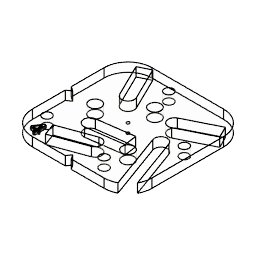
BearingPlate1_v15 (Autodesk Fusion 360 design; units mm, degrees)
Autodesk Fusion 360 part; units mm, degrees
derive "Sketch1" from "TopPlate v30"
sketch "sketch 220" plane through (0, 0, 0) normal (0, 0, 1) x (1, 0, 0)
  line L0 (55, -55) -> (-55, -55)
  line L1 (-55, -55) -> (-55, 55)
  line L2 (-55, 55) -> (55, 55)
  line L3 (55, 55) -> (55, -55)
  circle A0 centre (0, 9) radius 2
  circle A1 centre (0, -11) radius 1
  circle A2 centre (0, 0) radius 0.5
  circle A3 centre (-27, 47.000001) radius 3
  circle A4 centre (-1, 47.000001) radius 3
  circle A5 centre (46.868551, 27.224139) radius 3
  line L4 (46.998834, 0.999974) -> (46.985542, 27.034985) construction
  line L5 (-1, 47.000001) -> (-27, 47.000001) construction
  circle A6 centre (47.00084, 0.993878) radius 3
  circle A7 centre (-47.000001, -1) radius 3
  line L6 (-47.00798, -2.91748) -> (-47.001224, -28.99998) construction
  circle A8 centre (-47.000001, -27) radius 3
  circle A9 centre (0.015779, -47.131819) radius 3
  line L7 (1, -47.000001) -> (27, -47.000001) construction
  circle A10 centre (27.974555, -46.624476) radius 3
  line L8 (27.974555, -46.624476) -> (11, 0) construction
  line L9 (0, 0) -> (5, 0) construction
  line L10 (9.120675, -0.684205) -> (12.879325, 0.684205) construction
  line L11 (12.879325, 0.684205) -> (16.984556, -10.591746)
  line L12 (9.120675, -0.684205) -> (13.225906, -11.960156)
  line L13 (16.984556, -10.591746) -> (13.225906, -11.960156)
  circle A11 centre (11, 0) radius 2
  line L14 (-0.684205, -9.120675) -> (-11.960156, -13.225906)
  line L15 (-10.591746, -16.984556) -> (-11.960156, -13.225906)
  line L16 (0.684205, -12.879325) -> (-10.591746, -16.984556)
  circle A12 centre (0, -11) radius 2
  line L17 (-46.624476, -27.974555) -> (0, -11) construction
  circle A13 centre (7.778175, 7.778175) radius 2
  line L18 (7.778175, 7.778175) -> (46.868551, 27.224139) construction
  line L19 (7.778175, 7.778175) -> (8.668964, 5.987506) construction
  line L20 (8.668964, 5.987506) -> (19.412977, 11.33224)
  line L21 (19.412977, 11.33224) -> (17.631398, 14.913578)
  line L22 (17.631398, 14.913578) -> (6.887385, 9.568843)
  circle A14 centre (-7.778175, 7.778175) radius 2
  line L23 (-7.778175, 7.778175) -> (-27, 47.000001) construction
  line L24 (-7.778175, 7.778175) -> (-9.574099, 6.898028) construction
  line L25 (-9.574099, 6.898028) -> (-14.854975, 17.673572)
  line L26 (-5.982251, 8.658321) -> (-11.263127, 19.433864)
  line L27 (-11.263127, 19.433864) -> (-14.854975, 17.673572)
  line L28 (46.998834, 0.999974) -> (-6.363961, -6.363961) construction
  line L29 (0.015779, -47.131819) -> (-11, 0) construction
  line L30 (0, 9) -> (-47.00798, -2.91748) construction
  circle A15 centre (7.778175, -7.778175) radius 2
  line L31 (7.778175, -7.778175) -> (-1, 47.000001) construction
  line L32 (0, 0) -> (9, 0) construction
  circle A16 centre (-6.363961, -6.363961) radius 2
  line L33 (0, -11) -> (0.684205, -12.879325)
  circle A17 centre (-11, 0) radius 2
  line L34 (-11, 0) -> (-9.052486, 0.455178) construction
  line L35 (-9.052486, 0.455178) -> (-6.321415, -11.229908)
  line L36 (-6.321415, -11.229908) -> (-10.216444, -12.140265)
  line L37 (-10.216444, -12.140265) -> (-12.947514, -0.455178)
  line L38 (-6.363961, -6.363961) -> (-6.090557, -8.345185) construction
  line L39 (-6.090557, -8.345185) -> (5.79679, -6.704761)
  line L40 (5.79679, -6.704761) -> (5.249981, -2.742312)
  line L41 (5.249981, -2.742312) -> (-6.637365, -4.382737)
  line L42 (7.778175, -7.778175) -> (9.752979, -7.461713) construction
  line L43 (9.752979, -7.461713) -> (7.854211, 4.387113)
  line L44 (7.854211, 4.387113) -> (3.904602, 3.75419)
  line L45 (3.904602, 3.75419) -> (5.80337, -8.094636)
  line L46 (0, 9) -> (0.491492, 7.061331) construction
  line L47 (0.491492, 7.061331) -> (-11.140519, 4.11238)
  line L48 (-11.140519, 4.11238) -> (-12.123503, 7.989717)
  line L49 (-12.123503, 7.989717) -> (-0.491492, 10.938669)
  line L50 (20, -20) -> (-20, -20)
  line L51 (-20, -20) -> (-20, 20)
  line L52 (-20, 20) -> (20, 20)
  line L53 (20, 20) -> (20, -20)
  line L54 (20, -20) -> (-20, 20) construction
  line L55 (-20, -20) -> (20, 20) construction
  line L56 (15.105231, -11.275951) -> (11, 0) construction
  line L57 (13.052616, -5.637976) -> (14.931941, -4.95377) construction
  line L58 (13.052616, -5.637976) -> (11.17329, -6.322181) construction
  line L59 (14.931941, -4.95377) -> (17.281097, -4.098514) construction
  line L60 (16.767943, -2.68902) -> (17.794251, -5.508008)
  line L61 (17.794251, -5.508008) -> (9.337288, -8.586931)
  line L62 (16.767943, -2.68902) -> (8.31098, -5.767943)
  line L63 (8.31098, -5.767943) -> (9.337288, -8.586931)
  line L64 (18.522187, 13.122909) -> (7.778175, 7.778175) construction
  line L65 (13.150181, 10.450542) -> (14.04097, 8.659873) construction
  line L66 (14.04097, 8.659873) -> (15.154457, 6.421537) construction
  line L67 (13.811455, 5.753445) -> (16.497458, 7.089629)
  line L68 (13.811455, 5.753445) -> (9.802904, 13.811455)
  line L69 (9.802904, 13.811455) -> (12.488907, 15.147639)
  line L70 (12.488907, 15.147639) -> (16.497458, 7.089629)
  line L71 (-13.059051, 18.553718) -> (-7.778175, 7.778175) construction
  line L72 (-10.418613, 13.165946) -> (-6.377784, 15.146275) construction
  line L73 (-7.037894, 16.493218) -> (-5.717674, 13.799332)
  line L74 (-7.037894, 16.493218) -> (-5.717674, 13.799332) construction
  line L75 (-5.717674, 13.799332) -> (-13.799332, 9.838675)
  line L76 (-13.799332, 9.838675) -> (-15.119551, 12.532561)
  line L77 (-15.119551, 12.532561) -> (-7.037894, 16.493218)
  line L78 (0, 9) -> (-11.632011, 6.051048) construction
  line L79 (-5.816006, 7.525524) -> (-4.710149, 3.16352) construction
  line L80 (-6.16415, 2.794901) -> (-3.256147, 3.532139) construction
  line L81 (-3.256147, 3.532139) -> (-6.16415, 2.794901)
  line L82 (-6.16415, 2.794901) -> (-8.375864, 11.518909)
  line L83 (-8.375864, 11.518909) -> (-5.467861, 12.256147)
  line L84 (-5.467861, 12.256147) -> (-3.256147, 3.532139)
  line L85 (-11, 0) -> (-8.268929, -11.685087) construction
  line L86 (-9.634465, -5.842543) -> (-14.016372, -6.866695) construction
  line L87 (-14.357756, -5.406059) -> (-13.674988, -8.327331) construction
  line L88 (-14.357756, -5.406059) -> (-13.674988, -8.327331)
  line L89 (-13.674988, -8.327331) -> (-4.911173, -6.279028)
  line L90 (-4.911173, -6.279028) -> (-5.593941, -3.357756)
  line L91 (-5.593941, -3.357756) -> (-14.357756, -5.406059)
  line L92 (5.523385, -4.723536) -> (-6.363961, -6.363961) construction
  line L93 (-0.420288, -5.543749) -> (-1.035447, -1.085994) construction
  line L94 (-2.521365, -1.291047) -> (0.450471, -0.880941) construction
  line L95 (-2.521365, -1.291047) -> (0.450471, -0.880941)
  line L96 (0.450471, -0.880941) -> (1.68079, -9.796451)
  line L97 (1.68079, -9.796451) -> (-1.291047, -10.206557)
  line L98 (-1.291047, -10.206557) -> (-2.521365, -1.291047)
  line L99 (0, -11) -> (-11.275951, -15.105231) construction
  line L100 (-5.637976, -13.052616) -> (-4.098514, -17.281097) construction
  line L101 (-5.508008, -17.794251) -> (-2.68902, -16.767943) construction
  line L102 (-2.68902, -16.767943) -> (-5.508008, -17.794251)
  line L103 (-5.508008, -17.794251) -> (-8.586931, -9.337288)
  line L104 (-8.586931, -9.337288) -> (-5.767943, -8.31098)
  line L105 (-5.767943, -8.31098) -> (-2.68902, -16.767943)
  line L106 (7.778175, -7.778175) -> (5.879406, 4.070651) construction
  line L107 (6.82879, -1.853762) -> (11.2721, -1.141723) construction
  line L108 (11.034754, 0.33938) -> (11.509446, -2.622827) construction
  line L109 (11.034754, 0.33938) -> (11.509446, -2.622827)
  line L110 (11.509446, -2.622827) -> (2.622827, -4.046903)
  line L111 (2.622827, -4.046903) -> (2.148135, -1.084696)
  line L112 (2.148135, -1.084696) -> (11.034754, 0.33938)
  line L113 (0, -20) -> (0, -18.5) construction
  line L114 (0, -20) -> (1, -20) construction
  line L115 (0, -20) -> (-1, -20) construction
  line L116 (-1, -20) -> (0, -18.5)
  line L117 (1, -20) -> (0, -18.5)
  line L118 (-20, 0) -> (-18.5, 0) construction
  line L119 (-18.5, 0) -> (-20, 1)
  line L120 (-18.5, 0) -> (-20, -1)
  line L121 (-20, -1) -> (-20, 0) construction
  line L122 (-20, 0) -> (-20, 1) construction
  circle A18 centre (6, -14) radius 1.5
  circle A19 centre (16.104187, 2.735059) radius 1.5
  circle A20 centre (-2.329709, 15.997455) radius 1.5
  circle A21 centre (-15.675516, -11.444861) radius 1.5
  line L123 (-15.271796, -18.277941) -> (-12.271824, -18.255298) construction
  line L124 (-12.271824, -18.255298) -> (-12.301745, -14.291027) construction
  line L125 (-12.301745, -14.291027) -> (-15.301717, -14.313669) construction
  line L126 (-15.301717, -14.313669) -> (-15.271796, -18.277941) construction
extrude "Extrude1" add sketch "sketch 220" along normal blind 3 contours A0 | A0 L47 L49 L84 | A14 L26 L47 L49 L82 L84 | L26 L49 L83 L84 | L47 L81 L82 L84 | A14 L26 L49 L82 L83 | A14 L26 L49 | A14 L25 L47 L48 L49 L82 | A14 L49 L82 | A14 L25 L26 L49 L75 L82 L83 | A14 L49 L82 | A14 L49 L82 | L25 L26 L75 L77 | L26 L73 L75 L77 | A14 L49 L82 | A14 L25 L49 | L25 L26 L27 L77 | L25 L75 L76 L77 | A1 L97 | A1 A12 L33 L97 | A1 L97 | A1 A12 L97 L98 | A1 A12 L33 L97 L98 | L14 A12 L39 L96 L97 L98 | L14 L16 A12 L98 L105 | L14 A12 L98 | L16 L102 L103 L105 | L14 L16 L35 L36 L103 L105 | L14 A16 L35 L39 L98 L104 L105 | L39 L41 L45 L96 L110 L111 | L39 L41 L96 L98 | L14 L15 L16 L103 | L14 L35 L104 L105 | A16 L39 L41 L90 L98 | L39 L40 L45 L110 | A15 L39 L40 L43 L45 L62 L63 L110 | L41 L95 L96 L98 | L14 L36 L103 | L14 L35 L36 | L14 L35 L36 L103 L104 | A16 L35 L89 L90 | L41 L45 L110 L111 | L40 L41 L45 L110 | A15 L61 L63 | L41 L45 L111 L112 | A16 L35 L36 L37 L89 L103 L104 | A16 L35 L89 | A16 L41 L90 | A16 L35 L41 L90 L91 | L40 L41 L43 L45 L110 L112 | A15 L43 L62 L63 | A15 L61 L63 | L12 A15 L43 L61 L62 | A16 L35 L89 L90 | A16 L35 L37 L89 L91 | A16 L35 L89 | L12 L43 L62 L110 | L12 A11 L43 L110 L112 | L43 L44 L45 L112 | L11 L12 L13 L61 | L11 L12 L61 L62 | L37 L88 L89 L91 | A17 L35 L37 L91 | L11 L12 A11 L62 L109 L110 | L12 A11 L109 L110 | L11 L60 L61 L62 | A17 | A11 L109 L112 | A11 L109 L112 | A13 | A13 L20 L22 L68 | L22 L68 L69 L70 | L20 L22 L68 L70 | L20 L67 L68 L70 | L20 L21 L22 L70 | L50 L51 L52 L53 L116 L117 L119 L120 picked at (-1.219323, 9.210669) picked at (-3.564662, 8.147682) picked at (-4.838382, 7.931269) picked at (-6.443705, 11.149054) picked at (-5.399604, 3.848426) picked at (-7.839618, 11.011821) picked at (-6.458435, 9.358913) picked at (-10.94604, 6.333375) picked at (-7.145501, 7.044572) picked at (-9.614425, 10.627606) picked at (-7.781251, 9.547253) picked at (-7.864423, 6.890387) picked at (-11.237291, 13.321545) picked at (-7.654351, 13.963839) picked at (-7.962534, 9.534137) picked at (-9.927706, 8.286734) picked at (-11.140191, 16.153214) picked at (-12.742802, 11.470092) picked at (-0.071212, -10.70625) picked at (0.694181, -12.511167) picked at (-0.087629, -10.031035) picked at (-0.953643, -9.889262) picked at (-1.399257, -10.489014) picked at (-0.140921, -8.018037) picked at (-3.44742, -12.248834) picked at (-1.318461, -9.438021) picked at (-3.913768, -16.326994) picked at (-5.409652, -13.69793) picked at (-4.028443, -9.451367) picked at (3.182394, -6.033589) picked at (-1.006729, -4.951692) picked at (-10.094526, -13.965636) picked at (-6.05103, -10.18773) picked at (-2.732261, -5.858854) picked at (5.419133, -4.654291) picked at (7.299753, -4.141458) picked at (-1.416835, -1.979855) picked at (-7.421284, -11.529282) picked at (-6.471001, -11.246437) picked at (-7.417194, -9.798265) picked at (-5.848701, -7.059258) picked at (3.350068, -3.318512) picked at (5.097854, -3.059012) picked at (7.124082, -7.422643) picked at (4.014672, -2.199251) picked at (-10.014657, -9.745304) picked at (-7.901163, -7.076706) picked at (-5.575037, -4.400598) picked at (-6.753213, -3.889074) picked at (7.619057, -1.938971) picked at (8.778576, -5.697178) picked at (8.763172, -6.801763) picked at (10.699853, -6.702025) picked at (-6.110127, -5.837391) picked at (-10.507628, -6.272533) picked at (-7.968221, -6.896793) picked at (9.998801, -4.385203) picked at (9.360286, -2.193422) picked at (7.012366, 1.213932) picked at (13.965636, -10.094526) picked at (13.508006, -4.940076) picked at (-13.091113, -7.163916) picked at (-10.145587, -3.565463) picked at (12.196123, -3.693263) picked at (10.754963, -2.497921) picked at (15.886044, -5.138516) picked at (-11.989866, 0.33394) picked at (10.808606, -1.201245) picked at (9.686082, 0.219353) picked at (8.312655, 7.903069) picked at (11.068613, 9.395611) picked at (12.335897, 13.21002) picked at (13.894778, 10.07635) picked at (13.964465, 7.691064) picked at (15.539254, 12.383615) picked at (-18.373184, 11.17752)
fillet "Fillet1" radius 8 4 edges at (-20, -20, 1.5) (-20, 20, 1.5) (20, 20, 1.5) (20, -20, 1.5)
extrude "Extrude2" cut sketch "sketch 220" along normal blind 3 contours A0 | A14 L26 L49 L82 L83 | A14 L26 L49 | A14 L49 L82 | A14 L25 L26 L49 L75 L82 L83 | A14 L49 L82 | A14 L49 L82 | L25 L26 L75 L77 | A14 L49 L82 | A14 L25 L49 | L25 L26 L27 L77 | A1 L97 | A1 A12 L33 L97 | A1 L97 | A1 A12 L97 L98 | A1 A12 L33 L97 L98 | L14 L16 A12 L98 L105 | L14 A12 L98 | L14 L16 L35 L36 L103 L105 | L39 L41 L45 L96 L110 L111 | L39 L41 L96 L98 | L14 L15 L16 L103 | A16 L39 L41 L90 L98 | L39 L40 L45 L110 | L14 L35 L36 | A16 L35 L89 L90 | L41 L45 L110 L111 | L40 L41 L45 L110 | A15 L61 L63 | A16 L35 L89 | A16 L41 L90 | A15 L61 L63 | A16 L35 L89 L90 | A16 L35 L89 | L11 L12 L13 L61 | L11 L12 L61 L62 | L11 L12 A11 L62 L109 L110 | L12 A11 L109 L110 | A17 | A11 L109 L112 | A11 L109 L112 | A13 | A13 L20 L22 L68 | L20 L22 L68 L70 | L20 L21 L22 L70 picked at (-1.219323, 9.210669) picked at (-7.839618, 11.011821) picked at (-6.458435, 9.358913) picked at (-7.145501, 7.044572) picked at (-9.614425, 10.627606) picked at (-7.781251, 9.547253) picked at (-7.864423, 6.890387) picked at (-11.237291, 13.321545) picked at (-7.962534, 9.534137) picked at (-9.927706, 8.286734) picked at (-11.140191, 16.153214) picked at (-0.071212, -10.70625) picked at (0.694181, -12.511167) picked at (-0.087629, -10.031035) picked at (-0.953643, -9.889262) picked at (-1.399257, -10.489014) picked at (-3.44742, -12.248834) picked at (-1.318461, -9.438021) picked at (-5.409652, -13.69793) picked at (3.182394, -6.033589) picked at (-1.006729, -4.951692) picked at (-10.094526, -13.965636) picked at (-2.732261, -5.858854) picked at (5.419133, -4.654291) picked at (-6.471001, -11.246437) picked at (-5.848701, -7.059258) picked at (3.350068, -3.318512) picked at (5.097854, -3.059012) picked at (7.124082, -7.422643) picked at (-7.901163, -7.076706) picked at (-5.575037, -4.400598) picked at (8.763172, -6.801763) picked at (-6.110127, -5.837391) picked at (-7.968221, -6.896793) picked at (13.965636, -10.094526) picked at (13.508006, -4.940076) picked at (12.196123, -3.693263) picked at (10.754963, -2.497921) picked at (-11.989866, 0.33394) picked at (10.808606, -1.201245) picked at (9.686082, 0.219353) picked at (8.312655, 7.903069) picked at (11.068613, 9.395611) picked at (13.894778, 10.07635) picked at (15.539254, 12.383615)
extrude "Extrude3" cut 1 faces at (15.731673, -11.047883, 1) along direction (0.3421026, -0.9396626, 0) blind 9.5
sketch "Sketch1" plane through (0, 0, 3) normal (0, 0, 1) x (-1, 0, 0)
  line L0 (-12.879325, -0.684205) -> (-18.943713, 15.973015)
  arc A0 (-18.943713, 15.973015) -> (-20, 12) centre (-12, 12) ccw
  line L1 (-20, 12) -> (-20, -12)
  arc A1 (-20, -12) -> (-12, -20) centre (-12, -12) ccw
  line L2 (-12, -20) -> (12, -20)
  arc A2 (12, -20) -> (20, -12) centre (12, -12) ccw
  line L3 (20, -12) -> (20, -1)
  line L4 (20, -1) -> (18.5, 0)
  line L5 (18.5, 0) -> (20, 1)
  line L6 (20, 1) -> (20, 12)
  arc A3 (20, 12) -> (12, 20) centre (12, 12) ccw
  line L7 (12, 20) -> (1, 20)
  line L8 (1, 20) -> (0, 18.5)
  line L9 (0, 18.5) -> (-1, 20)
  line L10 (-1, 20) -> (-12, 20)
  arc A4 (-12, 20) -> (-15.802859, 19.038343) centre (-12, 12) ccw
  line L11 (-15.802859, 19.038343) -> (-9.120675, 0.684205)
  arc A5 (-12.879325, -0.684205) -> (-9.120675, 0.684205) centre (-11, 0) ccw
  circle A6 centre (0, -9) radius 2
  line L12 (9.574099, -6.898028) -> (14.854975, -17.673572)
  line L13 (14.854975, -17.673572) -> (11.263127, -19.433864)
  line L14 (11.263127, -19.433864) -> (5.982251, -8.658321)
  arc A7 (9.574099, -6.898028) -> (5.982251, -8.658321) centre (7.778175, -7.778175) ccw
  circle A8 centre (-7.778175, 7.778175) radius 2
  line L15 (-5.249981, 2.742312) -> (-5.79679, 6.704761)
  line L16 (-5.79679, 6.704761) -> (6.090557, 8.345185)
  arc A9 (6.637365, 4.382737) -> (6.090557, 8.345185) centre (6.363961, 6.363961) ccw
  line L17 (6.637365, 4.382737) -> (-5.249981, 2.742312)
  line L18 (-17.631398, -14.913578) -> (-19.412977, -11.33224)
  line L19 (-19.412977, -11.33224) -> (-8.668964, -5.987506)
  arc A10 (-6.887385, -9.568843) -> (-8.668964, -5.987506) centre (-7.778175, -7.778175) ccw
  line L20 (-6.887385, -9.568843) -> (-17.631398, -14.913578)
  line L21 (10.591746, 16.984556) -> (11.960156, 13.225906)
  line L22 (11.960156, 13.225906) -> (0.684205, 9.120675)
  arc A11 (-0.684205, 12.879325) -> (0.684205, 9.120675) centre (0, 11) ccw
  line L23 (-0.684205, 12.879325) -> (10.591746, 16.984556)
  circle A12 centre (11, 0) radius 2
  circle A13 centre (2.329709, -15.997455) radius 1.5
  circle A14 centre (15.675516, 11.444861) radius 1.5
  circle A15 centre (-16.104187, -2.735059) radius 1.5
  circle A16 centre (0, 0) radius 0.5
  circle A17 centre (-6, 14) radius 1.5
  line L24 (15.3, 18.3) -> (12.2, 18.3) construction
  line L25 (12.2, 18.3) -> (12.2, 14.3) construction
  line L26 (12.2, 14.3) -> (15.3, 14.3) construction
  line L27 (15.3, 14.3) -> (15.3, 18.3) construction
  dimension "d9" = 4
  dimension "d10" = 0
  text T0 "4" font "Arial" height 4 align left top in box 3.1 x 4 at (15.3, 18.3) x (-1, 0) y (0, -1) spacing 1 kerned
extrude "Extrude4" cut sketch "Sketch1" against normal blind 1 text T0
move_face "OffsetFaces1" offset -0.1 1 faces at (-13.094683, 14.081724, 1)
move_face "OffsetFaces2" offset -0.1 4 faces at (-8.201506, -11.857496, 2) (1.287533, -3.28912, 1) (14.050061, 13.132, 1) (11.348069, -6.802251, 1)
equation "d10 = '4'"
